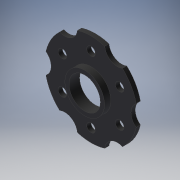
# Autodesk Inventor part: HELP_6204BEARING_CASE_B
Saved by Autodesk Inventor 2018 (Build 220112000, 112)
## iProperties
Created: 2026-07-04
Part Number: HELP_6204BEARING_CASE_B
Material: Generic
Document SubType Name: Modeling
Designer: neo
Density: 1 g/cm^3
Appearance: Default
Author: neo
Autodesk Inventor part; units mm, degrees
ref_plane "YZ Plane" through (0, 0, 0) normal (1, 0, 0) x (0, 1, 0)
ref_plane "XZ Plane" through (0, 0, 0) normal (0, 1, 0) x (-1, 0, 0)
ref_plane "XY Plane" through (0, 0, 0) normal (0, 0, 1) x (1, 0, 0)
sketch "Sketch1" plane through (0, 0, 0) normal (0, 1, 0) x (-1, 0, 0)
  circle A0 centre (0, 0) radius 18.5
  circle A1 centre (0, 0) radius 39 construction
  circle A2 centre (0, -39) radius 5.1
  circle A3 centre (0, 0) radius 54.5
  circle A4 centre (0, 0) radius 62 construction
  circle A5 centre (-62, 0) radius 15
  dimension "d1" = 78
  dimension "d11" = 124
  dimension "d0" = 37
  dimension "d2" = 10.2
  dimension "d3" = 109
  dimension "d12" = 30
  constraints: 4 centre point, 4 coincident, 1 horizontal alignment, 1 vertical alignment, 4 other
  measures "d0" diameter of A0
  measures "d2" diameter of A2
  measures "d3" diameter of A3
  measures "d12" diameter of A5
extrude "Extrusion1" add sketch "Sketch1" along normal blind 5 contours A2 | A3 A5 | A5 A3 picked at (16.1327, -31.6474) picked at (-51.8988, 0)
extrude "Extrusion2" cut sketch "Sketch1" along normal through all contours A2
pattern_circular "Circular Pattern1" count 6 over 360 about axis through (0, 0, 0) along (0, 1, 0) of "Extrusion2"
extrude "Extrusion3" cut sketch "Sketch1" along normal through all contours A5 A3 | A3 A5 picked at (-51.8988, 0) picked at (-61.8988, 0)
pattern_circular "Circular Pattern2" count 6 over 360 about axis through (0, 0, 0) along (0, 1, 0) of "Extrusion3"
sketch "Sketch2" plane through (0, 0, 0) normal (0, -1, 0) x (1, 0, 0)
  circle A0 centre (0, 0) radius 23.3
  circle A1 centre (0, 0) radius 18.5
  dimension "d18" = 46.6
  dimension "d19" = 37
  constraints: 2 centre point, 2 coincident
  measures "d18" diameter of A0
  measures "d19" diameter of A1
extrude "Extrusion4" add sketch "Sketch2" along normal blind 7.5
body "Solid1"
